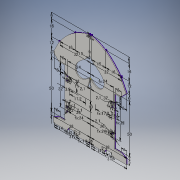
# Autodesk Inventor part: shitaita
Saved by Autodesk Inventor 2016 (Build 200138000, 138)
## iProperties
Created: 2016-08-31
Part Number: shitaita
Material: 一般
Document SubType Name: Modeling
Designer: KOTA-NPC2
Density: 1 g/cm^3
Appearance: 既定
Author: KOTA-NPC2
Autodesk Inventor part; units mm, degrees
ref_plane "YZ Plane" through (0, 0, 0) normal (1, 0, 0) x (0, 1, 0)
sketch "shitaita" plane through (0, 0, 0) normal (0, 0, 1) x (1, 0, 0)
  line L0 (-26, 0) -> (-26, -50)
  line L1 (26, 0) -> (26, -50)
  line L2 (-26, 0) -> (-32, 0)
  line L3 (32, 0) -> (38, 6)
  line L4 (-32, 0) -> (-38, 6)
  line L5 (-38, 6) -> (-32, 18)
  line L6 (38, 6) -> (32, 18)
  line L7 (26, 0) -> (32, 0)
  line L8 (-26, -50) -> (-32, -50)
  line L9 (-32, -50) -> (-38, -53)
  line L10 (-38, -53) -> (-38, -58)
  spline S0 degree 2 poles (-32, 18) (-18.1162, 37.2094) (-1, 40) knots 0 0 0 1 1 1
  spline S1 degree 2 poles (32, 18) (18.1162, 37.2094) (1, 40) knots 0 0 0 1 1 1
  line L11 (-1, 40) -> (0, 38)
  line L12 (0, 38) -> (1, 40)
  line L13 (26, -50) -> (32, -50)
  line L14 (32, -50) -> (38, -53)
  line L15 (38, -53) -> (38, -58)
  line L16 (-1, -58) -> (0, -56)
  line L17 (1, -58) -> (0, -56)
  circle A0 centre (-24, -9) radius 1.05
  circle A1 centre (-24, -41) radius 1.05
  circle A2 centre (24, -9) radius 1.05
  circle A3 centre (24, -41) radius 1.05
  line L18 (-22.1, -20) -> (-4.9, -20) construction
  line L19 (-4.9, -20) -> (-4.9, -30) construction
  line L20 (-4.9, -30) -> (-22.1, -30) construction
  line L21 (-22.1, -30) -> (-22.1, -20) construction
  line L22 (4.9, -20) -> (22.1, -20) construction
  line L23 (22.1, -20) -> (22.1, -30) construction
  line L24 (22.1, -30) -> (4.9, -30) construction
  line L25 (4.9, -30) -> (4.9, -20) construction
  line L26 (-25, -12.05) -> (-23, -12.05)
  line L27 (-23, -12.05) -> (-23, -14.15)
  line L28 (-23, -14.15) -> (-25, -14.15)
  line L29 (-25, -14.15) -> (-25, -12.05)
  line L30 (23, -12.05) -> (25, -12.05)
  line L31 (25, -12.05) -> (25, -14.15)
  line L32 (25, -14.15) -> (23, -14.15)
  line L33 (23, -14.15) -> (23, -12.05)
  line L34 (23, -35.85) -> (25, -35.85)
  line L35 (25, -35.85) -> (25, -37.95)
  line L36 (25, -37.95) -> (23, -37.95)
  line L37 (23, -37.95) -> (23, -35.85)
  line L38 (-25, -35.85) -> (-23, -35.85)
  line L39 (-23, -35.85) -> (-23, -37.95)
  line L40 (-23, -37.95) -> (-25, -37.95)
  line L41 (-25, -37.95) -> (-25, -35.85)
  line L42 (1, -58) -> (15, -58)
  line L43 (15, -58) -> (17, -55)
  line L44 (17, -55) -> (22, -55)
  line L45 (22, -55) -> (24, -58)
  line L46 (24, -58) -> (38, -58)
  line L47 (-1, -58) -> (-15, -58)
  line L48 (-38, -58) -> (-24, -58)
  line L49 (-24, -58) -> (-22, -55)
  line L50 (-22, -55) -> (-17, -55)
  line L51 (-17, -55) -> (-15, -58)
  point P0 (0, 0)
  point P1 (-16, 34)
  point P2 (16, 34)
  dimension "d35" = 50
  dimension "d37" = 26
  dimension "d38" = 26
  dimension "d39" = 6
  dimension "d44" = 6
  dimension "d45" = 6
  dimension "d46" = 6
  dimension "d48" = 6
  dimension "d49" = 6
  dimension "d50" = 12
  dimension "d51" = 32
  dimension "d52" = 12
  dimension "d53" = 32
  dimension "d56" = 32
  dimension "d57" = 32
  dimension "d59" = 38
  dimension "d61" = 3
  dimension "d65" = 6
  dimension "d66" = 16
  dimension "d67" = 15
  dimension "d68" = 16
  dimension "d69" = 6
  dimension "d70" = 16
  dimension "d71" = 15
  dimension "d72" = 6
  dimension "d73" = 16
  dimension "d74" = 2
  dimension "d75" = 1
  dimension "d81" = 6
  dimension "d82" = 38
  dimension "d83" = 3
  dimension "d84" = 50
  dimension "d85" = 37
  dimension "d86" = 37
  dimension "d87" = 2
  dimension "d88" = 2
  dimension "d89" = 5
  dimension "d90" = 1
  dimension "d113" = 2.1
  dimension "d114" = 2.1
  dimension "d115" = 2.1
  dimension "d116" = 2.1
  dimension "d117" = 24
  dimension "d118" = 24
  dimension "d119" = 24
  dimension "d120" = 24
  dimension "d121" = 32
  dimension "d122" = 32
  dimension "d123" = 9
  dimension "d124" = 9
  dimension "d127" = 10
  dimension "d128" = 17.2
  dimension "d129" = 17.2
  dimension "d130" = 3.9
  dimension "d131" = 3.9
  dimension "d132" = 11
  dimension "d135" = 1
  dimension "d136" = 2
  dimension "d137" = 2
  dimension "d138" = 2.1
  dimension "d139" = 1
  dimension "d140" = 2
  dimension "d141" = 2
  dimension "d142" = 2.1
  constraints: 104 end point, 14 parallel, 13 horizontal, 7 perpendicular, 5 point on line, 4 centre point, 3 vertical, 1 collinear, 6 other
  measures "d35" distance of L0.start L0.end
  measures "d37" distance from line of point (0, 0) L1
  measures "d38" distance from line of L0 point (0, 0)
  measures "d39" distance of L0.start L2.end
  measures "d44" distance of L1.start L3.start
  measures "d45" horizontal distance of L3.start L3.end
  measures "d46" horizontal distance of L3.start L3.end
  measures "d48" horizontal distance of L2.end L4.end
  measures "d49" horizontal distance of L2.end L4.end
  measures "d50" vertical distance of L4.end L5.end
  measures "d51" horizontal distance of point (0, 0) L5.end
  measures "d52" vertical distance of L3.end L6.end
  measures "d53" horizontal distance of point (0, 0) L6.end
  measures "d56" distance of point (0, 0) L3.start
  measures "d57" distance of point (0, 0) L2.end
  measures "d59" horizontal distance of point (0, 0) L9.end
  measures "d61" vertical distance of L8.end L9.end
  measures "d65" horizontal distance of L8.end L9.end
  measures "d66" horizontal distance of L5.end point (-16, 34)
  measures "d67" horizontal distance of point (-16, 34) L11.start
  measures "d68" horizontal distance of L5.end point (-16, 34)
  measures "d69" vertical distance of point (-16, 34) L11.start
  measures "d70" horizontal distance of L6.end point (16, 34)
  measures "d71" horizontal distance of L12.end point (16, 34)
  measures "d72" vertical distance of point (16, 34) L12.end
  measures "d73" horizontal distance of L6.end point (16, 34)
  measures "d74" vertical distance of L11.end L11.start
  measures "d75" horizontal distance of L11.end L11.start
  measures "d81" horizontal distance of L13.end L14.end
  measures "d82" horizontal distance of L14.end point (0, 0)
  measures "d83" vertical distance of L13.end L14.end
  measures "d84" vertical distance of point (0, 0) L1.end
  measures "d85" distance of L10.end L16.start
  measures "d86" distance of L15.end L17.start
  measures "d87" vertical distance of L17.start L16.end
  measures "d88" vertical distance of L16.start L16.end
  measures "d89" distance of L14.end L15.end
  measures "d90" horizontal distance of L16.end L16.start
  measures "d113" diameter of A0
  measures "d114" diameter of A1
  measures "d115" diameter of A2
  measures "d116" diameter of A3
  measures "d117" horizontal distance of point (0, 0) A0.centre
  measures "d118" horizontal distance of point (0, 0) A1.centre
  measures "d119" horizontal distance of point (0, 0) A2.centre
  measures "d120" horizontal distance of A3.centre point (0, 0)
  measures "d121" distance of A1.centre A0.centre
  measures "d122" distance of A3.centre A2.centre
  measures "d123" vertical distance of point (0, 0) A2.centre
  measures "d124" vertical distance of point (0, 0) A0.centre
  measures "d127" distance of L20.end L18.start
  measures "d128" distance of L18.start L18.end
  measures "d129" distance of L22.start L22.end
  measures "d130" distance between parallel lines of L0 L21
  measures "d131" distance between parallel lines of L1 L23
  measures "d132" distance from line of L18 A0.centre
  measures "d135" distance between parallel lines of L29 L0
  measures "d136" distance between parallel lines of L27 L29
  measures "d137" distance edge to line of A0 L26
  measures "d138" distance of L26.end L27.end
  measures "d139" distance between parallel lines of L0 L41
  measures "d140" distance of L39.end L40.end
  measures "d141" distance edge to line of A1 L40
  measures "d142" distance between parallel lines of L40 L38
sketch "肉抜き" plane through (0, 0, 0) normal (0, 0, 1) x (1, 0, 0)
  line L0 (-18, 27.0037) -> (-7, 23)
  line L1 (-7, 23) -> (-3, 23)
  line L2 (-3, 3) -> (-23.604, 3.005)
  line L3 (-23.604, 3.005) -> (-28, 15.0921)
  line L4 (-28, 15.0921) -> (-18, 27.0037)
  line L5 (3, 3) -> (23.585, 2.9479)
  line L6 (23.585, 2.9479) -> (28, 14.9831)
  line L7 (28, 14.9831) -> (18, 26.9621)
  line L8 (18, 26.9621) -> (7, 22.9899)
  line L9 (7, 22.9899) -> (3, 23.0001)
  line L10 (-3, 23) -> (-3, 3)
  line L11 (3, 23.0001) -> (3, 3)
  point P0 (0, 0)
  dimension "d91" = 20
  dimension "d92" = 3
  dimension "d93" = 24
  dimension "d95" = 15
  dimension "d96" = 3
  dimension "d97" = 160
  dimension "d98" = 120
  dimension "d99" = 110
  dimension "d100" = 3
  dimension "d101" = 15
  dimension "d102" = 3
  dimension "d103" = 160
  dimension "d104" = 24
  dimension "d105" = 20
  dimension "d107" = 120
  dimension "d108" = 110
  dimension "d159" = 6
  dimension "d171" = 25
  dimension "d172" = 25
  dimension "d173" = 11
  dimension "d174" = 11
  constraints: 24 end point, 1 horizontal, 1 parallel, 1 vertical
  measures "d91" distance of L1.end L2.start
  measures "d92" horizontal distance of point (0, 0) L2.start
  measures "d93" distance from line of L2 L0.start
  measures "d95" horizontal distance of L1.end L0.start
  measures "d96" horizontal distance of point (0, 0) L2.start
  measures "d97" angle of L1 L0
  measures "d98" angle of L3 L4
  measures "d99" angle of L2 L3
  measures "d100" horizontal distance of point (0, 0) L5.start
  measures "d101" horizontal distance of L9.end L7.end
  measures "d102" horizontal distance of point (0, 0) L5.start
  measures "d103" angle of L9 L8
  measures "d104" distance from line of L5 L7.end
  measures "d105" distance between parallel lines of L5 L9
  measures "d107" angle of L6 L7
  measures "d108" angle of L5 L6
  measures "d159" distance of L9.end L1.end
  measures "d171" distance from line of L10 L3.end
  measures "d172" distance from line of L11 L6.end
  measures "d173" horizontal distance of L0.end L0.start
  measures "d174" horizontal distance of L8.end L7.end
ref_plane "作業平面1" through (0, 0, 0.5) normal (0, 0, 1) x (1, 0, 0)
sketch "スペード" plane through (0, 0, 0.5) normal (0, 0, 1) x (1, 0, 0)
  spline S0 degree 4 poles (0, 22) (-1.4423, 17.6996) (-12.6116, 11.4671) (-21.1598, 4.3372) (-9.9497, -8.6913) (-1, 1) knots 0 0 0 0 0 0.484032 1 1 1 1 1
  spline S1 degree 4 poles (0, 22) (1.4423, 17.6996) (12.6116, 11.4671) (21.1598, 4.3372) (9.9497, -8.6913) (1, 1) knots 0 0 0 0 0 0.484032 1 1 1 1 1
  spline S2 degree 2 poles (1, 1) (-0.3472, -2.0827) (2.5, -8) knots 0 0 0 1 1 1
  spline S3 degree 2 poles (-1, 1) (0.3472, -2.0827) (-2.5, -8) knots 0 0 0 1 1 1
  line L0 (-2.5, -8) -> (2.5, -8)
  circle A0 centre (0, 25) radius 1
  point P0 (0, 0)
  point P1 (-5, 16)
  point P2 (-12, 10)
  point P3 (-15, 4)
  point P4 (5, 16)
  point P5 (12, 10)
  point P6 (15, 4)
  point P7 (-13, -2)
  point P8 (13, -2)
  point P9 (0.6, -2)
  point P10 (-0.6, -2)
  dimension "d180" = 5
  dimension "d181" = 5
  dimension "d182" = 12
  dimension "d183" = 12
  dimension "d184" = 15
  dimension "d185" = 15
  dimension "d186" = 13
  dimension "d187" = 13
  dimension "d188" = 21
  dimension "d189" = 21
  dimension "d190" = 6
  dimension "d191" = 0
  dimension "d192" = 6
  dimension "d193" = 1
  dimension "d194" = 1
  dimension "d195" = 6
  dimension "d196" = 6
  dimension "d197" = 6
  dimension "d198" = 6
  dimension "d199" = 6
  dimension "d200" = 6
  dimension "d202" = 22
  dimension "d203" = 0.6
  dimension "d204" = 2.5
  dimension "d206" = 0.6
  dimension "d207" = 2.5
  dimension "d208" = 9
  dimension "d209" = 3
  dimension "d210" = 3
  dimension "d252" = 2
  dimension "d253" = 3
  dimension "d254" = 0
  constraints: 2 end point, 1 centre point, 1 horizontal, 18 other
  measures "d180" horizontal distance of point (0, 0) point (-5, 16)
  measures "d181" horizontal distance of point (0, 0) point (5, 16)
  measures "d182" horizontal distance of point (0, 0) point (-12, 10)
  measures "d183" horizontal distance of point (0, 0) point (12, 10)
  measures "d184" horizontal distance of point (0, 0) point (-15, 4)
  measures "d185" horizontal distance of point (0, 0) point (15, 4)
  measures "d186" horizontal distance of point (0, 0) point (-13, -2)
  measures "d187" horizontal distance of point (0, 0) point (13, -2)
  measures "d188" vertical distance of point (-1, 1) point (0, 22)
  measures "d189" vertical distance of point (1, 1) point (0, 22)
  measures "d190" vertical distance of point (-5, 16) point (0, 22)
  measures "d191" horizontal distance of point (0, 0) point (0, 22)
  measures "d192" vertical distance of point (0, 22) point (5, 16)
  measures "d193" horizontal distance of point (0, 0) point (-1, 1)
  measures "d194" horizontal distance of point (0, 0) point (1, 1)
  measures "d195" vertical distance of point (12, 10) point (5, 16)
  measures "d196" vertical distance of point (-5, 16) point (-12, 10)
  measures "d197" vertical distance of point (-15, 4) point (-12, 10)
  measures "d198" vertical distance of point (15, 4) point (12, 10)
  measures "d199" vertical distance of point (-13, -2) point (-15, 4)
  measures "d200" vertical distance of point (13, -2) point (15, 4)
  measures "d202" distance of point (0, 0) point (0, 22)
  measures "d203" horizontal distance of point (0, 0) point (0.6, -2)
  measures "d204" horizontal distance of L0.end point (0, 0)
  measures "d206" horizontal distance of point (0, 0) point (-0.6, -2)
  measures "d207" horizontal distance of point (0, 0) L0.start
  measures "d208" distance from line of L0 point (-1, 1)
  measures "d209" vertical distance of point (1, 1) point (0.6, -2)
  measures "d210" vertical distance of point (-0.6, -2) point (-1, 1)
  measures "d252" diameter of A0
  measures "d253" distance of point (0, 22) A0.centre
  measures "d254" horizontal distance of point (0, 22) A0.centre
ref_plane "作業平面3" through (0, 0, 0.5) normal (0, 0, 1) x (1, 0, 0)
sketch "スケッチ13" plane through (0, 0, 0.5) normal (0, 0, 1) x (1, 0, 0)
  spline S0 degree 2 poles (-2.5, -8) (0.3472, -2.0827) (-1, 1) knots 0 0 0 1 1 1 projected
  spline S1 degree 4 poles (-1, 1) (-9.9497, -8.6913) (-21.1598, 4.3372) (-12.6116, 11.4671) (-1.4423, 17.6996) (0, 22) knots 0 0 0 0 0 0.515968 1 1 1 1 1 projected
  spline S2 degree 4 poles (0, 22) (1.4423, 17.6996) (12.6116, 11.4671) (21.1598, 4.3372) (9.9497, -8.6913) (1, 1) knots 0 0 0 0 0 0.484032 1 1 1 1 1 projected
  spline S3 degree 2 poles (1, 1) (-0.3472, -2.0827) (2.5, -8) knots 0 0 0 1 1 1 projected
  line L0 (2.5, -8) -> (-2.5, -8) projected
  line L1 (22.1, -20) -> (22.1, -30) projected
  line L2 (22.1, -30) -> (4.9, -30) projected
  line L3 (4.9, -30) -> (4.9, -20) projected
  line L4 (4.9, -20) -> (22.1, -20) projected
  line L5 (-4.9, -20) -> (-4.9, -30) projected
  line L6 (-4.9, -30) -> (-22.1, -30) projected
  line L7 (-22.1, -30) -> (-22.1, -20) projected
  line L8 (-22.1, -20) -> (-4.9, -20) projected
  line L9 (-23, -35.85) -> (-23, -37.95) projected
  line L10 (-23, -37.95) -> (-25, -37.95) projected
  line L11 (-25, -37.95) -> (-25, -35.85) projected
  line L12 (-25, -35.85) -> (-23, -35.85) projected
  line L13 (25, -35.85) -> (25, -37.95) projected
  line L14 (25, -37.95) -> (23, -37.95) projected
  line L15 (23, -37.95) -> (23, -35.85) projected
  line L16 (23, -35.85) -> (25, -35.85) projected
  line L17 (25, -12.05) -> (25, -14.15) projected
  line L18 (25, -14.15) -> (23, -14.15) projected
  line L19 (23, -14.15) -> (23, -12.05) projected
  line L20 (23, -12.05) -> (25, -12.05) projected
  line L21 (-23, -12.05) -> (-23, -14.15) projected
  line L22 (-23, -14.15) -> (-25, -14.15) projected
  line L23 (-25, -14.15) -> (-25, -12.05) projected
  line L24 (-25, -12.05) -> (-23, -12.05) projected
  circle A0 centre (24, -41) radius 1.05 projected
  circle A1 centre (24, -9) radius 1.05 projected
  circle A2 centre (-24, -41) radius 1.05 projected
  circle A3 centre (-24, -9) radius 1.05 projected
  line L25 (-26, 0) -> (-26, -50) projected
  line L26 (-26, -50) -> (-32, -50) projected
  line L27 (-32, -50) -> (-38, -53) projected
  line L28 (-38, -53) -> (-38, -58) projected
  line L29 (-38, -58) -> (-24, -58) projected
  line L30 (-24, -58) -> (-22, -55) projected
  line L31 (-22, -55) -> (-17, -55) projected
  line L32 (-17, -55) -> (-15, -58) projected
  line L33 (-15, -58) -> (-1, -58) projected
  line L34 (-1, -58) -> (0, -56) projected
  line L35 (0, -56) -> (1, -58) projected
  line L36 (1, -58) -> (15, -58) projected
  line L37 (15, -58) -> (17, -55) projected
  line L38 (17, -55) -> (22, -55) projected
  line L39 (22, -55) -> (24, -58) projected
  line L40 (24, -58) -> (38, -58) projected
  line L41 (38, -58) -> (38, -53) projected
  line L42 (38, -53) -> (32, -50) projected
  line L43 (32, -50) -> (26, -50) projected
  line L44 (26, -50) -> (26, 0) projected
  line L45 (26, 0) -> (32, 0) projected
  line L46 (32, 0) -> (38, 6) projected
  line L47 (38, 6) -> (32, 18) projected
  spline S4 degree 2 poles (32, 18) (18.1162, 37.2094) (1, 40) knots 0 0 0 1 1 1 projected
  line L48 (1, 40) -> (0, 38) projected
  line L49 (0, 38) -> (-1, 40) projected
  spline S5 degree 2 poles (-1, 40) (-18.1162, 37.2094) (-32, 18) knots 0 0 0 1 1 1 projected
  line L50 (-32, 18) -> (-38, 6) projected
  line L51 (-38, 6) -> (-32, 0) projected
  line L52 (-32, 0) -> (-26, 0) projected
  point P0 (0, 0)
  constraints: 6 other
extrude "押し出し9" add sketch "スケッチ13" along normal mid plane 1 contours L1 L2 L3 L4 | L5 L6 L7 L8 | L52 L51 L50 S5 L49 L48 S4 L47 L46 L45 L44 L43 L42 L41 L40 L39 L38 L37 L36 L35 L34 L33 L32 L31 L30 L29 L28 L27 L26 L25
sketch "スケッチ17" plane through (0, 0, 0) normal (0, 0, -1) x (-1, 0, 0)
  line L0 (-17.57, -18.1972) -> (17.4001, -18.1972) construction
  line L1 (17.4001, -18.1972) -> (17.4001, -47.2973) construction
  line L2 (17.4001, -47.2973) -> (-17.57, -47.2973) construction
  line L3 (-17.57, -47.2973) -> (-17.57, -18.1972) construction
  point P0 (0, 0)
  constraints: 2 other
extrude "押し出し10" cut sketch "スペード" along normal mid plane 1 contours A0
